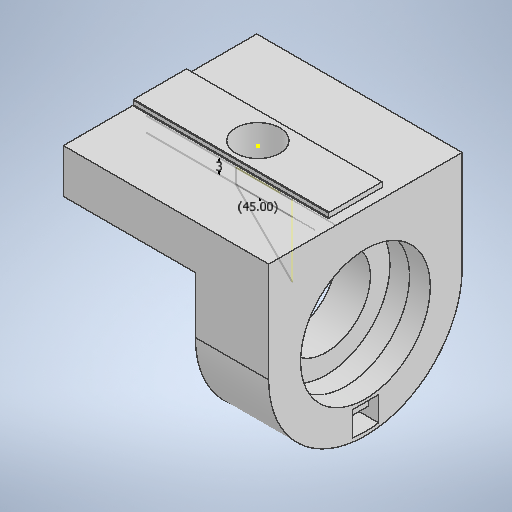
# Autodesk Inventor part: Base_Mount_Standard
Saved by Autodesk Inventor 2026.2 (Build 302298000, 298)
## iProperties
Created: 2026-03-23
Part Number: Base_Mount_Standard
Material: Generic
Document SubType Name: Modeling
Designer: Paco Ariel
Density: 1 g/cm^3
Appearance: Default
Author: Paco Ariel
Autodesk Inventor part; units mm, degrees
ref_plane "YZ Plane" through (0, 0, 0) normal (1, 0, 0) x (0, 1, 0)
ref_plane "XZ Plane" through (0, 0, 0) normal (0, 1, 0) x (-1, 0, 0)
ref_plane "XY Plane" through (0, 0, 0) normal (0, 0, 1) x (1, 0, 0)
sketch "Sketch1" plane through (0, 0, 0) normal (0, 1, 0) x (-1, 0, 0)
  line L0 (20, 19.775) -> (-20, 19.775)
  line L1 (-20, 19.775) -> (-20, -19.775)
  line L2 (-20, -19.775) -> (20, -19.775)
  line L3 (20, -19.775) -> (20, 19.775)
  line L4 (20, 19.775) -> (-20, -19.775) construction
  line L5 (-20, 19.775) -> (20, -19.775) construction
  circle A0 centre (0, 0) radius 4.5
  line L6 (-32.3892, 5.5) -> (32.3892, 5.5)
  line L7 (32.3892, 5.5) -> (32.3892, -5.5)
  line L8 (32.3892, -5.5) -> (-32.3892, -5.5)
  line L9 (-32.3892, -5.5) -> (-32.3892, 5.5)
  line L10 (-32.3892, 5.5) -> (32.3892, -5.5) construction
  line L11 (32.3892, 5.5) -> (-32.3892, -5.5) construction
  point P0 (-20, -5.5)
  point P1 (20, -5.5)
  point P2 (20, 5.5)
  point P3 (-20, 5.5)
  dimension "d0" = 40
  dimension "d1" = 39.55
  dimension "d2" = 9
  dimension "d3" = 11
  constraints: 24 end point, 4 midpoint, 4 parallel, 2 horizontal, 2 perpendicular, 1 centre point, 1 coincident
  measures "d0" distance of L2.end L1.end
  measures "d1" distance of L1.end L0.end
  measures "d2" diameter of A0
  measures "d3" distance of L6.end L7.end
extrude "Extrusion1" add sketch "Sketch1" along normal blind 1 contours L3 L8 L1 L6
extrude "Extrusion2" add sketch "Sketch1" against normal blind 6 contours L3 L6 L1 L0 | L3 L8 L1 L6 | L3 L2 L1 L8
fillet "Fillet1" radius 0.1 4 edges at (0, 0, 5.5) (0, 1, 5.5) (0, 1, -5.5) (0, 0, -5.5)
sketch "Sketch3" plane through (20, -6, 19.775) normal (1, 0, 0) x (0, 0, -1)
  line L0 (0, 6) -> (14.175, 6) projected
  line L1 (0, 6) -> (0, 0) projected
  circle A0 centre (19.775, -14.5) radius 13.25
  line L2 (0, -14.5) -> (0, 6)
  line L3 (0, 6) -> (39.55, 6)
  line L4 (39.55, 6) -> (39.55, -14.5)
  line L5 (19.775, -14.5) -> (19.775, 6)
  arc A1 (0, -14.5) -> (39.55, -14.5) centre (19.775, -14.5) ccw
  line L6 (19.775, 6) -> (19.775, -28.343)
  line L7 (22.4675, -28.343) -> (17.0825, -28.343)
  line L8 (22.4675, -28.343) -> (22.4675, -33.343)
  line L9 (17.0825, -28.343) -> (17.0825, -33.343)
  arc A2 (17.0825, -33.343) -> (22.4675, -33.343) centre (19.775, -14.5) ccw
  line L10 (22.4675, -31.343) -> (17.0825, -31.343)
  dimension "d12" = 26.5
  dimension "d13" = 20.5
  dimension "d15" = 39.55
  dimension "d17" = 19.775
  dimension "d18" = 34.343
  dimension "d19" = 5.385
  dimension "d20" = 5
  dimension "d22" = 3
  constraints: 18 end point, 4 point on circle, 3 centre point, 3 vertical, 2 coincident, 2 perpendicular, 2 point on line, 1 horizontal, 1 midpoint, 1 parallel, 1 tangent
  measures "d12" diameter of A0
  measures "d13" distance of L5.start L5.end
  measures "d15" distance of L0.start L3.end
  measures "d17" radius of A1
  measures "d18" distance of L5.end L6.end
  measures "d19" distance of L7.start L7.end
  measures "d20" distance of L8.end L7.start
  measures "d22" distance between parallel lines of L10 L7
extrude "Extrusion3" add sketch "Sketch3" along normal blind 2
extrude "Extrusion4" add sketch "Sketch3" against normal blind 6 contours L0 L3 L4 A1 L2 L1 | L8 L10 L9 L7
sketch "Sketch4" plane through (14, -6, 19.775) normal (-1, 0, 0) x (0, 0, 1)
  circle A0 centre (-19.775, -14.5) radius 13.25 projected
  circle A1 centre (-19.775, -14.5) radius 13
  point P0 (-19.775, 6)
  dimension "d27" = 26
  constraints: 1 centre point, 1 coincident
  measures "d27" diameter of A1
extrude "Extrusion5" add sketch "Sketch4" against normal blind 4
chamfer "Chamfer1" distance 0.25 distance2 4 1 edges at (18, -20.5, 13.25) measured on face at (18, -20.5, 13.15)
sketch "Sketch5" plane through (14, -6, 19.775) normal (-1, 0, 0) x (0, 0, 1)
  circle A0 centre (-19.775, -14.5) radius 13 projected
  circle A1 centre (-19.775, -14.5) radius 9
  arc A2 (-39.55, -14.5) -> (0, -14.5) centre (-19.775, -14.5) ccw
  line L0 (0, -14.5) -> (0, 0) projected
  line L1 (-39.55, 0) -> (-39.55, -14.5) projected
  line L2 (0, 0) -> (-39.55, 0) projected
  point P0 (-19.775, 6)
  dimension "d33" = 18
  constraints: 2 centre point, 2 coincident, 2 end point, 2 point on circle
  measures "d33" diameter of A1
extrude "Extrusion6" add sketch "Sketch5" along normal blind 7 contours A0 | L1 L2 L0 A2
extrude "Extrusion7" cut sketch "Sketch3" against normal through all contours L8 A2 L9 L10
sketch "Sketch2" plane through (0, -6, 0) normal (0, -1, 0) x (1, 0, 0)
  circle A0 centre (0, 0) radius 7
  line L0 (-20, 19.775) -> (-20, -19.775) projected
  line L1 (20, 19.775) -> (-20, 19.775) projected
  line L2 (-20, -19.775) -> (20, -19.775) projected
  line L3 (7, 19.775) -> (7, -19.775) projected
  point P0 (7, 0)
  dimension "d8" = 14
  constraints: 1 centre point, 1 coincident
  measures "d8" diameter of A0
sketch "Sketch6" plane through (0, 0, 0) normal (0, 0, 1) x (1, 0, 0)
  line L0 (4.5, -6) -> (-4.5, -6) projected
  line L1 (-4.5, -6) -> (16.0061, -6) construction
  line L2 (7, -6) -> (7, -20.5) projected
  line L3 (7, -6) -> (-22.7644, -6)
  line L4 (7, -9) -> (-22.7644, -9)
  line L5 (-4.5, -6) -> (-4.5, -9)
  line L6 (-4.5, -9) -> (7, -20.5)
  line L7 (-4.5, -9) -> (11.7635, -9) construction
  point P0 (0, 0)
  dimension "d39" = 3
  dimension "d40" = 45
  constraints: 12 end point, 3 horizontal, 1 equal length, 1 parallel, 1 perpendicular, 1 point on line
  measures "d39" distance between parallel lines of L3 L4
  measures "d40" angle of L6 L7
extrude "Extrusion8" add sketch "Sketch2" along normal blind 3
body "Solid1"
